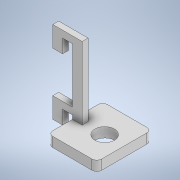
# Autodesk Inventor part: round_0_5_inchHoleV01
Saved by Autodesk Inventor 2020.2 (Build 242310000, 310)
## iProperties
Created: 2020-03-08
Part Number: round_0_5_inchHoleV01
Material: Generic
Document SubType Name: Modeling
Designer: robst
Density: 1 g/cm^3
Appearance: Default
Author: robst
Autodesk Inventor part; units mm, degrees
ref_plane "YZ Plane" through (0, 0, 0) normal (1, 0, 0) x (0, 1, 0)
ref_plane "XZ Plane" through (0, 0, 0) normal (0, 1, 0) x (-1, 0, 0)
ref_plane "XY Plane" through (0, 0, 0) normal (0, 0, 1) x (1, 0, 0)
sketch "Sketch1" plane through (0, 0, 0) normal (0, 0, 1) x (1, 0, 0)
  line L0 (0, 6.35) -> (0, 53.34)
  line L1 (0, 53.34) -> (-19.05, 53.34)
  line L2 (-19.05, 53.34) -> (-19.05, 55.245)
  line L3 (-12.7, 48.895) -> (-6.35, 48.895)
  line L4 (-6.35, 48.895) -> (-6.35, 13.335)
  line L5 (-6.35, 13.335) -> (-19.05, 13.335)
  line L6 (-19.05, 13.335) -> (-19.05, 12.7)
  line L7 (-12.7, 8.89) -> (-6.35, 8.89)
  line L8 (-6.35, 8.89) -> (-6.35, 0)
  line L9 (-6.35, 0) -> (0, 0)
  line L10 (-19.05, 55.245) -> (-19.05, 40.005)
  line L11 (-19.05, 40.005) -> (-12.7, 40.005)
  line L12 (-12.7, 40.005) -> (-12.7, 48.895)
  line L13 (-19.05, 12.7) -> (-19.05, 0)
  line L14 (-19.05, 0) -> (-12.7, 0)
  line L15 (-12.7, 0) -> (-12.7, 8.89)
  line L16 (0, 0) -> (0, 6.35)
  point P0 (-19.05, 53.34)
  point P1 (-19.05, 11.43)
  dimension "d1" = 35.56
  dimension "d2" = 4.445
  dimension "d3" = 4.445
  dimension "d4" = 6.35
  dimension "d6" = 6.35
  dimension "d7" = 6.35
  dimension "d13" = 13.335
  dimension "d14" = 13.335
  constraints: 34 end point, 9 perpendicular, 4 point on line, 3 vertical, 1 collinear, 1 parallel
  measures "d1" distance of L3.end L4.end
  measures "d2" distance between parallel lines of L5 L7
  measures "d3" distance between parallel lines of L1 L3
  measures "d4" distance between parallel lines of L4 L0
  measures "d6" distance between parallel lines of L12 L4
  measures "d7" distance between parallel lines of L10 L12
  measures "d13" distance between parallel lines of L11 L1
  measures "d14" distance between parallel lines of L5 L14
extrude "Extrusion1" add sketch "Sketch1" along normal mid plane 3.81
sketch "Sketch4" plane through (0, 0, 0) normal (0, 0, 1) x (1, 0, 0)
  line L0 (0, 0) -> (-6.35, 0) projected
  line L1 (-6.35, 0) -> (25.4, 0)
  line L2 (25.4, 0) -> (25.4, 6.35)
  line L3 (25.4, 6.35) -> (-6.35, 6.35)
  line L4 (-6.35, 6.35) -> (-6.35, 0)
  dimension "d23" = 31.75
  dimension "d24" = 6.35
  constraints: 8 end point, 2 parallel, 1 horizontal, 1 perpendicular
  measures "d23" distance of L3.end L2.end
  measures "d24" distance of L2.end L1.end
extrude "Extrusion4" add sketch "Sketch4" against normal mid plane 35.56
sketch "Sketch5" plane through (-6.35, 6.35, 17.78) normal (0, 1, 0) x (1, 0, 0)
  line L0 (31.75, 35.56) -> (0, 35.56) construction
  line L1 (6.35, 35.56) -> (6.35, 0) construction
  line L2 (31.75, 0) -> (0, 0) construction
  line L3 (31.75, 35.56) -> (31.75, 0) construction
  line L4 (6.35, 35.56) -> (31.75, 0) construction
  line L5 (31.75, 0) -> (6.35, 0) construction
  line L6 (31.75, 35.56) -> (6.35, 0) construction
  circle A0 centre (19.05, 17.78) radius 6.35
  point P0 (6.35, 17.78)
  dimension "d27" = 12.7
  constraints: 8 end point, 2 point on line, 1 centre point, 1 midpoint, 1 perpendicular, 1 vertical
  measures "d27" diameter of A0
extrude "Extrusion5" cut sketch "Sketch5" against normal through all
fillet "Fillet2" radius 3.175 4 edges at (-6.35, 3.175, 17.78) (25.4, 3.175, 17.78) (25.4, 3.175, -17.78) (-6.35, 3.175, -17.78)
equation "\"d11\" = width"
equation "\"width\" = 3.81"
body "Solid1"
